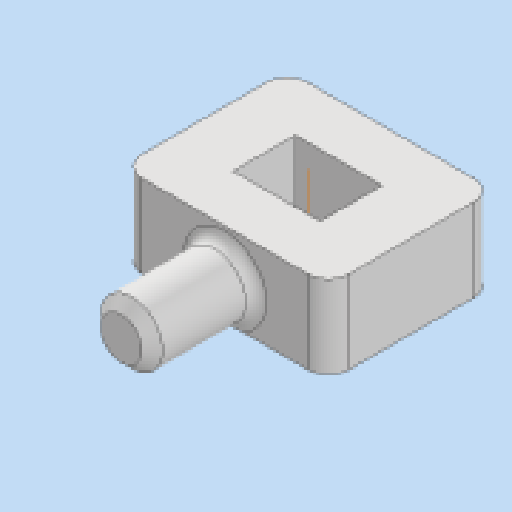
# Autodesk Inventor part: Pen_nib_stopper
Saved by Autodesk Inventor 2024 (Build 280153000, 153)
## iProperties
Created: 2025-02-15
Part Number: Pen_nib_stopper
Material: Generic
Document SubType Name: Modeling
Designer: XxPan
Density: 1 g/cm^3
Appearance: Default
Author: XxPan
Autodesk Inventor part; units mm, degrees
ref_plane "YZ Plane" through (0, 0, 0) normal (1, 0, 0) x (0, 1, 0)
ref_plane "XZ Plane" through (0, 0, 0) normal (0, 1, 0) x (-1, 0, 0)
ref_plane "XY Plane" through (0, 0, 0) normal (0, 0, 1) x (1, 0, 0)
sketch "Sketch1" plane through (0, 0, 0) normal (0, 1, 0) x (-1, 0, 0)
  line L0 (2.1, 1.5) -> (-2.1, 1.5)
  line L1 (-2.1, -1.5) -> (2.1, -1.5)
  line L2 (7, 0) -> (-7, 0) construction
  line L3 (0, -5.6) -> (0, 5.6) construction
  line L4 (5, 4) -> (-5, 4)
  line L5 (-5, 4) -> (-5, -4)
  line L6 (-5, -4) -> (5, -4)
  line L7 (5, -4) -> (5, 4)
  line L8 (-2, 0.84) -> (-2, -0.76) projected
  line L9 (2, -0.76) -> (2, 0.84) projected
  line L10 (-2.1, 1.5) -> (-2.1, -1.5)
  line L11 (2.1, -1.5) -> (2.1, 1.5)
  line L12 (0.2, 1.5) -> (-0.2, 1.5) projected
  point P0 (0, 0)
  point P1 (2.3, 0)
  point P2 (0, 1.5)
  dimension "d2" = 3
  dimension "d3" = 10
  dimension "d16" = 2.5
  dimension "d17" = 2.5
  dimension "d29" = 0.1
  dimension "d30" = 0.1
  constraints: 16 end point, 5 parallel, 2 horizontal, 2 point on line, 1 collinear, 1 midpoint, 1 perpendicular, 1 other
  measures "d2" distance of L1.start L0.end
  measures "d3" distance of L6.end L5.end
  measures "d16" distance between parallel lines of L0 L4
  measures "d17" distance between parallel lines of L1 L6
  measures "d29" distance between parallel lines of L8 L10
  measures "d30" distance between parallel lines of L9 L11
extrude "Extrusion1" add sketch "Sketch1" along normal blind 4
sketch "Sketch2" plane through (-5, 0, 4) normal (0, 0, 1) x (1, 0, 0)
  circle A0 centre (5, 1.8) radius 1.5
  line L0 (0, 4) -> (10, 4) construction
  line L1 (5, -1.76) -> (5, 10.56) construction
  line L2 (0, 0) -> (0, 4) projected
  arc A1 (7, 8.5082) -> (3, 8.5082) centre (5, 1.8) ccw projected
  point P0 (5, 0)
  point P1 (0, 2)
  dimension "d7" = 3
  constraints: 1 centre point, 1 coincident, 1 midpoint, 1 point on line
  measures "d7" diameter of A0
extrude "Extrusion2" add sketch "Sketch2" along normal blind 5
sketch "Sketch4" plane through (5, 0, -4) normal (0, 0, -1) x (-1, 0, 0)
  circle A0 centre (5, 1.8) radius 0.2 construction
  circle A1 centre (5, 1.8) radius 0.5
  line L0 (4.6464, 2.1536) -> (5, 2.5071)
  line L1 (5, 2.5071) -> (5.3536, 2.1536)
  point P0 (5, 0)
  dimension "d18" = 1
  constraints: 4 end point, 2 point on circle, 2 tangent, 1 centre point, 1 coincident, 1 perpendicular, 1 vertical alignment
  measures "d18" diameter of A1
extrude "Extrusion4" cut sketch "Sketch4" against normal blind 1
chamfer "Chamfer2" distance 0.2 angle 45 3 edges at (-0.1768, 2.3303, -4) (0, 1.3, -4) (0.1768, 2.3303, -4)
chamfer "Chamfer3" distance 0.5 angle 45 1 edges at (-1.5, 1.8, 9)
fillet "Fillet1" radius 0.5 1 edges at (-1.5, 1.8, 4)
fillet "Fillet2" radius 1 4 edges at (-5, 2, 4) (-5, 2, -4) (5, 2, -4) (5, 2, 4)
body "Solid1"
